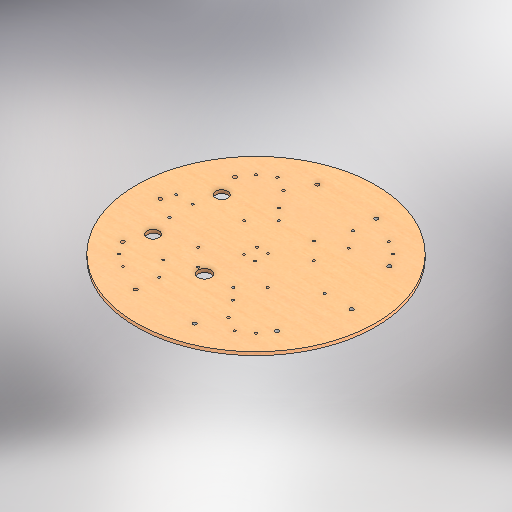
# Autodesk Inventor part: layer2
Saved by Autodesk Inventor 2026 (Build 300175050, 175E)
## iProperties
Created: 2025-06-05
Part Number: layer2
Material: Generic
Document SubType Name: Modeling
Designer: satom
Density: 1 g/cm^3
Appearance: Default
Author: satom
Autodesk Inventor part; units mm, degrees
ref_plane "YZ Plane" through (0, 0, 0) normal (1, 0, 0) x (0, 1, 0)
ref_plane "XZ Plane" through (0, 0, 0) normal (0, 1, 0) x (-1, 0, 0)
ref_plane "XY Plane" through (0, 0, 0) normal (0, 0, 1) x (1, 0, 0)
sketch "Sketch1" plane through (0, 0, 0) normal (0, 1, 0) x (-1, 0, 0)
  arc A0 (0, -177) -> (0, 177) centre (0, 0) ccw
  arc A1 (0, 177) -> (0, -177) centre (0, 0) ccw
  point P0 (-177, 177)
  point P1 (-177, -177)
  dimension "d0" = 354
  constraints: 4 point on circle, 2 centre point, 2 coincident
  measures "d0" diameter of A0
extrude "Extrusion1" add sketch "Sketch1" along normal blind 5
sketch "Sketch2" plane through (0, 5, 0) normal (0, 1, 0) x (1, 0, 0)
  circle A0 centre (-51.435, -34.125) radius 1.7
  circle A1 centre (-51.435, 34.125) radius 1.7
  circle A2 centre (51.435, 34.125) radius 1.7
  circle A3 centre (51.435, -34.125) radius 1.7
  line L0 (151.6, 177) -> (0, 177) construction
  line L1 (0, -177) -> (0, 177) construction
  circle A4 centre (0, 0) radius 177 construction
  line L2 (-177, 0) -> (177, 0) construction
  circle A5 centre (26.035, 59.5249) radius 1.7
  circle A6 centre (26.035, -59.5249) radius 1.7
  circle A7 centre (-26.035, 59.5249) radius 1.7
  circle A8 centre (-26.035, -59.5249) radius 1.7
  point P0 (177, 177)
  dimension "d5" = 3.4
  dimension "d6" = 3.4
  dimension "d8" = 3.4
  dimension "d10" = 3.4
  dimension "d12" = 68.25
  dimension "d13" = 68.25
  dimension "d14" = 102.87
  dimension "d15" = 102.87
  dimension "d18" = 51.435
  dimension "d19" = 51.435
  dimension "d20" = 34.125
  dimension "d21" = 34.125
  dimension "d153" = 3.4
  dimension "d155" = 3.4
  dimension "d157" = 3.4
  dimension "d159" = 3.4
  dimension "d161" = 52.07
  dimension "d162" = 26.035
  dimension "d163" = 52.07
  dimension "d164" = 26.035
  dimension "d165" = 119.0498
  dimension "d166" = 119.0498
  dimension "d167" = 59.5249
  dimension "d168" = 59.5249
  constraints: 8 centre point, 4 end point, 1 horizontal, 1 point on circle, 1 vertical
  measures "d5" diameter of A0
  measures "d6" diameter of A1
  measures "d8" diameter of A2
  measures "d10" diameter of A3
  measures "d12" distance of A2.centre A3.centre
  measures "d13" distance of A1.centre A0.centre
  measures "d14" distance of A3.centre A0.centre
  measures "d15" distance of A1.centre A2.centre
  measures "d18" distance from line of L1 A3.centre
  measures "d19" distance from line of L1 A2.centre
  measures "d20" distance from line of L2 A0.centre
  measures "d21" distance from line of L2 A3.centre
  measures "d153" diameter of A5
  measures "d155" diameter of A6
  measures "d157" diameter of A7
  measures "d159" diameter of A8
  measures "d161" distance of A5.centre A7.centre
  measures "d162" distance from line of L1 A5.centre
  measures "d163" distance of A8.centre A6.centre
  measures "d164" distance from line of L1 A6.centre
  measures "d165" distance of A5.centre A6.centre
  measures "d166" distance of A8.centre A7.centre
  measures "d167" distance from line of L2 A6.centre
  measures "d168" distance from line of L2 A8.centre
extrude "Jetson Holes" cut sketch "Sketch2" against normal through all
sketch "Sketch3" plane through (0, 5, 0) normal (0, 1, 0) x (1, 0, 0)
  circle A0 centre (-12.7, -63.5) radius 9.525
  circle A1 centre (0, 0) radius 177 construction
  line L0 (151.6, 177) -> (0, 177) construction
  line L1 (-177, 0) -> (0, 0) construction
  line L2 (0, 0) -> (0, -177) construction
  point P0 (177, 177)
  dimension "d24" = 19.05
  dimension "d189" = 63.5
  dimension "d190" = 12.7
  constraints: 4 end point, 2 point on circle, 1 centre point, 1 vertical
  measures "d24" diameter of A0
  measures "d189" distance from line of L1 A0.centre
  measures "d190" distance from line of A0.centre L2
extrude "SPI_Holes" cut sketch "Sketch3" against normal through all
sketch "Sketch4" plane through (0, 5, 0) normal (0, 1, 0) x (1, 0, 0)
  circle A0 centre (-60.96, -76.2) radius 1.7
  circle A1 centre (60.96, -101.6) radius 1.7
  circle A2 centre (60.96, 76.2) radius 1.7
  circle A3 centre (-60.96, 101.6) radius 1.7
  line L0 (177, 0) -> (-177, 0) construction
  circle A4 centre (-12.7, -63.5) radius 9.525 construction
  circle A5 centre (-101.6, 50.8) radius 8.89
  circle A6 centre (-101.6, -50.8) radius 8.89
  circle A7 centre (41.91, -76.2) radius 1.7
  circle A8 centre (-41.91, -101.6) radius 1.7
  circle A9 centre (-41.91, 76.2) radius 1.7
  circle A10 centre (41.91, 101.6) radius 1.7
  point P0 (0, 0)
  point P1 (0, -177)
  dimension "d30" = 3.4
  dimension "d31" = 3.4
  dimension "d33" = 3.4
  dimension "d35" = 3.4
  dimension "d37" = 121.92
  dimension "d38" = 121.92
  dimension "d39" = 25.4
  dimension "d40" = 25.4
  dimension "d43" = 12.7
  dimension "d44" = 177.8
  dimension "d45" = 17.78
  dimension "d46" = 17.78
  dimension "d47" = 50.8
  dimension "d48" = 50.8
  dimension "d139" = 3.4
  dimension "d140" = 19.05
  dimension "d141" = 25.4
  dimension "d142" = 3.4
  dimension "d143" = 19.05
  dimension "d144" = 25.4
  dimension "d145" = 3.4
  dimension "d147" = 3.4
  dimension "d149" = 25.4
  dimension "d150" = 25.4
  dimension "d151" = 19.05
  dimension "d152" = 19.05
  constraints: 10 centre point, 2 end point, 1 horizontal
  measures "d30" diameter of A0
  measures "d31" diameter of A1
  measures "d33" diameter of A2
  measures "d35" diameter of A3
  measures "d37" horizontal distance of A2.centre A3.centre
  measures "d38" horizontal distance of A1.centre A0.centre
  measures "d39" vertical distance of A3.centre A2.centre
  measures "d40" vertical distance of A1.centre A0.centre
  measures "d43" vertical distance of A4.centre A0.centre
  measures "d44" distance of A2.centre A1.centre
  measures "d45" diameter of A5
  measures "d46" diameter of A6
  measures "d47" distance from line of L0 A5.centre
  measures "d48" distance from line of L0 A6.centre
  measures "d139" diameter of A7
  measures "d140" horizontal distance of A1.centre A7.centre
  measures "d141" vertical distance of A1.centre A7.centre
  measures "d142" diameter of A8
  measures "d143" horizontal distance of A0.centre A8.centre
  measures "d144" vertical distance of A0.centre A8.centre
  measures "d145" diameter of A9
  measures "d147" diameter of A10
  measures "d149" vertical distance of A2.centre A10.centre
  measures "d150" vertical distance of A3.centre A9.centre
  measures "d151" horizontal distance of A2.centre A10.centre
  measures "d152" horizontal distance of A3.centre A9.centre
extrude "NiMH Holes" cut sketch "Sketch4" against normal through all
sketch "Sketch5" plane through (0, 5, 0) normal (0, 1, 0) x (1, 0, 0)
  circle A0 centre (-8.1625, 9.55) radius 1.7
  circle A1 centre (-8.1625, -9.55) radius 1.7
  circle A2 centre (8.1625, -9.55) radius 1.7
  circle A3 centre (8.1625, 9.55) radius 1.7
  line L0 (-177, 0) -> (177, 0)
  line L1 (0, 177) -> (0, -177) construction
  circle A4 centre (0, 0) radius 177 construction
  dimension "d53" = 3.4
  dimension "d54" = 3.4
  dimension "d56" = 3.4
  dimension "d58" = 3.4
  dimension "d60" = 16.325
  dimension "d61" = 16.325
  dimension "d62" = 19.1
  dimension "d63" = 19.1
  dimension "d66" = 9.55
  dimension "d67" = 9.55
  dimension "d191" = 8.1625
  dimension "d192" = 8.1625
  constraints: 4 centre point, 4 end point, 1 point on circle, 1 vertical
  measures "d53" diameter of A0
  measures "d54" diameter of A1
  measures "d56" diameter of A2
  measures "d58" diameter of A3
  measures "d60" distance of A3.centre A0.centre
  measures "d61" distance of A2.centre A1.centre
  measures "d62" distance of A0.centre A1.centre
  measures "d63" distance of A2.centre A3.centre
  measures "d66" distance from line of L0 A1.centre
  measures "d67" distance from line of L0 A2.centre
  measures "d191" distance from line of L1 A0.centre
  measures "d192" distance from line of L1 A1.centre
extrude "IMU Holes" cut sketch "Sketch5" against normal through all
sketch "Sketch8" plane through (0, 5, 0) normal (0, 1, 0) x (1, 0, 0)
  circle A0 centre (-101.6, 101.6) radius 1.7
  circle A1 centre (-101.6, -101.6) radius 1.7
  circle A2 centre (101.6, -101.6) radius 1.7
  circle A3 centre (101.6, 101.6) radius 1.7
  line L0 (177, -151.6) -> (177, 151.6) construction
  line L1 (177, 0) -> (-177, 0) construction
  circle A4 centre (0, 0) radius 177 construction
  line L2 (151.6, 177) -> (0, 177) construction
  line L3 (0, -177) -> (151.6, -177) construction
  line L4 (0, 177) -> (0, -177) construction
  circle A5 centre (101.6, 0) radius 1.7
  point P0 (177, -177)
  point P1 (177, 177)
  dimension "d97" = 3.4
  dimension "d98" = 3.4
  dimension "d100" = 3.4
  dimension "d102" = 3.4
  dimension "d104" = 101.6
  dimension "d105" = 101.6
  dimension "d106" = 101.6
  dimension "d107" = 101.6
  dimension "d108" = 101.6
  dimension "d109" = 101.6
  dimension "d110" = 101.6
  dimension "d111" = 101.6
  dimension "d169" = 3.4
  dimension "d170" = 101.6
  constraints: 5 centre point, 4 end point, 1 horizontal, 1 midpoint, 1 point on circle, 1 point on line, 1 vertical
  measures "d97" diameter of A0
  measures "d98" diameter of A1
  measures "d100" diameter of A2
  measures "d102" diameter of A3
  measures "d104" distance from line of L4 A0.centre
  measures "d105" distance from line of L1 A0.centre
  measures "d106" distance from line of L1 A1.centre
  measures "d107" distance from line of L4 A1.centre
  measures "d108" distance from line of L4 A3.centre
  measures "d109" distance from line of L4 A2.centre
  measures "d110" distance from line of L1 A3.centre
  measures "d111" distance from line of L1 A2.centre
  measures "d169" diameter of A5
  measures "d170" distance from line of L4 A5.centre
extrude "Level1 Standoffs" cut sketch "Sketch8" against normal through all
sketch "Sketch6" plane through (0, 5, 0) normal (0, 1, 0) x (1, 0, 0)
  circle A0 centre (-82.55, -114.3) radius 1.7
  circle A1 centre (-82.55, 114.3) radius 1.7
  circle A2 centre (82.55, 114.3) radius 1.7
  circle A3 centre (82.55, -114.3) radius 1.7
  circle A4 centre (0, 0) radius 177 construction
  line L0 (177, -151.6) -> (177, 151.6) construction
  line L1 (0, -177) -> (151.6, -177) construction
  line L2 (0, 178.2067) -> (0, -177) construction
  line L3 (-177, 0) -> (177, 0) construction
  point P0 (0, 177)
  point P1 (177, -177)
  point P2 (177, 177)
  dimension "d70" = 3.4
  dimension "d71" = 3.4
  dimension "d73" = 3.4
  dimension "d75" = 3.4
  dimension "d77" = 82.55
  dimension "d80" = 82.55
  dimension "d81" = 82.55
  dimension "d84" = 82.55
  dimension "d85" = 114.3
  dimension "d86" = 114.3
  dimension "d87" = 114.3
  dimension "d88" = 114.3
  constraints: 4 centre point, 4 end point, 1 midpoint, 1 point on circle, 1 vertical
  measures "d70" diameter of A0
  measures "d71" diameter of A1
  measures "d73" diameter of A2
  measures "d75" diameter of A3
  measures "d77" distance from line of L2 A0.centre
  measures "d80" distance from line of L2 A1.centre
  measures "d81" distance from line of L2 A3.centre
  measures "d84" distance from line of L2 A2.centre
  measures "d85" distance from line of L3 A0.centre
  measures "d86" distance from line of L3 A1.centre
  measures "d87" distance from line of L3 A3.centre
  measures "d88" distance from line of L3 A2.centre
extrude "Level3 Standoffs" cut sketch "Sketch6" against normal through all
sketch "Sketch7" plane through (0, 5, 0) normal (0, 1, 0) x (1, 0, 0)
  line L0 (177, 0) -> (-177, 0) construction
  circle A0 centre (0, 0) radius 177 construction
  circle A1 centre (-141.44, 0) radius 2.667
  circle A2 centre (-114.4274, -83.1363) radius 2.667
  circle A3 centre (-114.4274, 83.1363) radius 2.667
  circle A4 centre (-43.7074, -134.5174) radius 2.667
  circle A5 centre (-43.7074, 134.5174) radius 2.667
  line L1 (0, 177) -> (0, -181.7127) construction
  circle A6 centre (141.44, 0) radius 2.667
  circle A7 centre (114.4274, -83.1363) radius 2.667
  circle A8 centre (114.4274, 83.1363) radius 2.667
  circle A9 centre (43.7074, -134.5174) radius 2.667
  circle A10 centre (43.7074, 134.5174) radius 2.667
  point P0 (-177, 0)
  point P1 (177, 0)
  dimension "d91" = 5.334
  dimension "d92" = 35.56
  dimension "d95" = 144
  constraints: 10 centre point, 7 symmetric about line, 4 end point, 3 point on circle, 1 horizontal, 1 point on line, 1 vertical, 14 other
  measures "d91" diameter of A1
  measures "d92" distance of A0.end A1.centre
extrude "Zip Ties" cut sketch "Sketch7" against normal through all
sketch "Sketch9" plane through (0, 5, 0) normal (0, 1, 0) x (1, 0, 0)
  circle A0 centre (-110.89, 17.1) radius 1.7
  circle A1 centre (-110.89, -17.1) radius 1.7
  circle A2 centre (-135.09, 17.1) radius 1.7
  line L0 (0, 0) -> (-177, 0) construction
  circle A3 centre (0, 0) radius 177 construction
  circle A4 centre (-141.44, 0) radius 2.667 construction
  point P0 (0, 177)
  point P1 (0, -177)
  dimension "d171" = 3.4
  dimension "d172" = 3.4
  dimension "d174" = 3.4
  dimension "d176" = 24.2
  dimension "d177" = 34.2
  dimension "d178" = 17.1
  dimension "d179" = 6.35
  dimension "d180" = 17.1
  dimension "d181" = 17.1
  constraints: 3 centre point, 2 end point, 1 horizontal, 1 point on circle
  measures "d171" diameter of A0
  measures "d172" diameter of A1
  measures "d174" diameter of A2
  measures "d176" distance of A0.centre A2.centre
  measures "d177" distance of A1.centre A0.centre
  measures "d178" distance from line of L0 A0.centre
  measures "d179" horizontal distance of A4.centre A2.centre
  measures "d180" distance from line of L0 A2.centre
  measures "d181" distance from line of L0 A1.centre
extrude "Mic_MCU_Case" cut sketch "Sketch9" against normal blind 25.4
equation "\"d0\" = robot_diameter"
equation "\"d3\" = hardboard_thickness"
equation "\"d5\" = m3_clearance"
equation "\"d6\" = d7"
equation "\"d8\" = d9"
equation "\"d10\" = d11"
equation "\"d13\" = d12"
equation "\"d19\" = d18"
equation "\"d20\" = d21"
equation "\"d21\" = 0.5 * d12"
equation "\"d153\" = d154"
equation "\"d155\" = d156"
equation "\"d157\" = d158"
equation "\"d159\" = d160"
equation "\"d162\" = 0.5 * d161"
equation "\"d163\" = d161"
equation "\"d164\" = d162"
equation "\"d166\" = d165"
equation "\"d167\" = 0.5 * d165"
equation "\"d168\" = d167"
equation "\"d30\" = m3_clearance"
equation "\"d31\" = d32"
equation "\"d33\" = d34"
equation "\"d35\" = d36"
equation "\"d38\" = d37"
equation "\"d40\" = d39"
equation "\"d46\" = d45"
equation "\"d48\" = d47"
equation "\"d139\" = m3_clearance"
equation "\"d141\" = d40"
equation "\"d142\" = m3_clearance"
equation "\"d144\" = d40"
equation "\"d145\" = d146"
equation "\"d147\" = d148"
equation "\"d149\" = d39"
equation "\"d150\" = d39"
equation "\"d152\" = d151"
equation "\"d53\" = m3_clearance"
equation "\"d54\" = d55"
equation "\"d56\" = d57"
equation "\"d58\" = d59"
equation "\"d61\" = d60"
equation "\"d63\" = d62"
equation "\"d66\" = 0.5 * d63"
equation "\"d67\" = d66"
equation "\"d97\" = m3_clearance"
equation "\"d98\" = d99"
equation "\"d100\" = d101"
equation "\"d102\" = d103"
equation "\"d106\" = d105"
equation "\"d107\" = d104"
equation "\"d108\" = d104"
equation "\"d109\" = d104"
equation "\"d110\" = d105"
equation "\"d111\" = d105"
equation "\"d169\" = m3_clearance"
equation "\"d70\" = m3_clearance"
equation "\"d71\" = d72"
equation "\"d73\" = d74"
equation "\"d75\" = d76"
equation "\"d80\" = d77"
equation "\"d81\" = d77"
equation "\"d84\" = d77"
equation "\"d86\" = d85"
equation "\"d87\" = d85"
equation "\"d88\" = d85"
equation "\"d171\" = m3_clearance"
equation "\"d172\" = d173"
equation "\"d174\" = d175"
equation "\"d178\" = 0.5 * d177"
equation "\"d180\" = d178"
equation "\"d181\" = d178"
equation "\"m3_heat_set_insert\" = 4"
equation "\"m3_clearance\" = 3.4"
equation "\"m3_heat_set_depth\" = 7"
equation "\"robot_diameter\" = 354"
equation "\"hardboard_thickness\" = 5"
equation "\"motor_centerline_height\" = 13"
equation "\"d7\" = 3.4"
equation "\"d9\" = 3.4"
equation "\"d11\" = 3.4"
equation "\"d154\" = 3.4"
equation "\"d156\" = 3.4"
equation "\"d158\" = 3.4"
equation "\"d160\" = 3.4"
equation "\"d32\" = 3.4"
equation "\"d34\" = 3.4"
equation "\"d36\" = 3.4"
equation "\"d146\" = 3.4"
equation "\"d148\" = 3.4"
equation "\"d55\" = 3.4"
equation "\"d57\" = 3.4"
equation "\"d59\" = 3.4"
equation "\"d99\" = 3.4"
equation "\"d101\" = 3.4"
equation "\"d103\" = 3.4"
equation "\"d72\" = 3.4"
equation "\"d74\" = 3.4"
equation "\"d76\" = 3.4"
equation "\"d173\" = 3.4"
equation "\"d175\" = 3.4"
body "Solid1"
